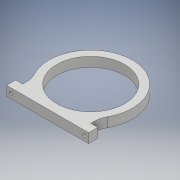
# Autodesk Inventor part: reservoir pump combo mount
Saved by Autodesk Inventor 2018 (Build 220112000, 112)
## iProperties
Created: 2018-06-16
Part Number: reservoir pump combo mount
Material: Generic
Document SubType Name: Modeling
Designer: John Viljoen
Density: 1 g/cm^3
Appearance: Default
Author: John Viljoen
Autodesk Inventor part; units mm, degrees
ref_plane "YZ Plane" through (0, 0, 0) normal (1, 0, 0) x (0, 1, 0)
ref_plane "XZ Plane" through (0, 0, 0) normal (0, 1, 0) x (-1, 0, 0)
ref_plane "XY Plane" through (0, 0, 0) normal (0, 0, 1) x (1, 0, 0)
sketch "Sketch1" plane through (0, 0, 0) normal (0, 0, 1) x (1, 0, 0)
  line L0 (0, 0) -> (72.4, 0)
  line L1 (72.4, 0) -> (72.4, 8)
  line L2 (72.4, 8) -> (0, 8)
  line L3 (0, 8) -> (0, 0)
  line L4 (36.2, 8) -> (36.2, 38) construction
  circle A0 centre (36.2, 38) radius 30
  circle A1 centre (36.2, 38) radius 36.75
  line L5 (6.2, 8) -> (6.2, 16.7735)
  line L6 (66.2, 8) -> (66.2, 16.7735)
  dimension "d0" = 72.4
  dimension "d1" = 8
  dimension "d2" = 30
  dimension "d3" = 60
  dimension "d4" = 73.5
  constraints: 14 end point, 3 parallel, 2 centre point, 2 coincident, 2 point on circle, 2 point on line, 2 vertical, 1 horizontal, 1 midpoint, 1 perpendicular
  measures "d0" distance of L2.end L1.end
  measures "d1" distance of L1.end L0.end
  measures "d2" distance of L4.start L4.end
  measures "d3" diameter of A0
  measures "d4" diameter of A1
extrude "Extrusion1" add sketch "Sketch1" along normal blind 8.4
fillet "Fillet1" radius 20 2 edges at (66.2, 16.7735, 4.2) (6.2, 16.7735, 4.2)
sketch "Sketch2" plane through (0, 0, 0) normal (0, -1, 0) x (1, 0, 0)
  line L0 (72.4, 0) -> (72.4, 8.4) projected
  line L1 (0, 0) -> (0, 8.4) construction
  line L2 (0, 4.2) -> (3.7, 4.2) construction
  circle A0 centre (3.7, 4.2) radius 1.5
  line L3 (72.4, 4.2) -> (68.7, 4.2) construction
  circle A1 centre (68.7, 4.2) radius 1.5
  dimension "d8" = 3.7
  dimension "d9" = 3
  dimension "d10" = 3.7
  dimension "d11" = 3
  constraints: 4 end point, 2 centre point, 2 coincident, 2 horizontal, 2 midpoint
  measures "d8" distance of L2.start L2.end
  measures "d9" diameter of A0
  measures "d10" distance of L3.start L3.end
  measures "d11" diameter of A1
extrude "Extrusion2" cut sketch "Sketch2" against normal up to surface (8 mm away)
body "Solid1"
